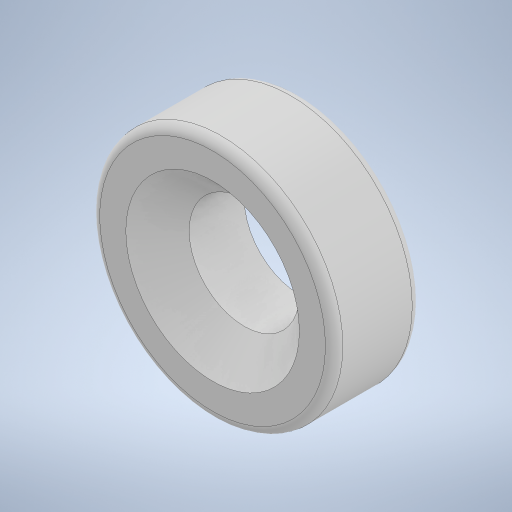
# Autodesk Inventor part: plate
Saved by Autodesk Inventor 2023 (Build 270158000, 158)
## iProperties
Created: 2023-07-16
Part Number: plate
Material: Generic
Document SubType Name: Modeling
Designer: checo
Density: 1 g/cm^3
Appearance: Default
Author: checo
Autodesk Inventor part; units mm, degrees
ref_plane "YZ Plane" through (0, 0, 0) normal (1, 0, 0) x (0, 1, 0)
ref_plane "XZ Plane" through (0, 0, 0) normal (0, 1, 0) x (-1, 0, 0)
ref_plane "XY Plane" through (0, 0, 0) normal (0, 0, 1) x (1, 0, 0)
sketch "Sketch1" plane through (0, 0, 0) normal (0, 0, 1) x (1, 0, 0)
  circle A0 centre (0, 0) radius 7
  dimension "d0" = 14
  constraints: 2 coincident, 1 centre point
  measures "d0" diameter of A0
extrude "Extrusion1" add sketch "Sketch1" against normal blind 5
hole "Hole1" at (0, 0, 0) direction (0, 0, -1) diameter 6.35 end through all countersink diameter 10 countersink angle 90
fillet "Fillet1" radius 0.5 2 edges at (-7, 0, 0) (-7, 0, -5)
body "Solid1"
